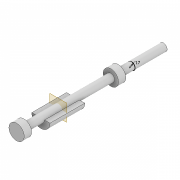
# Autodesk Inventor part: балансирный_вал
Saved by Autodesk Inventor 2021 (Build 250183000, 183)
## iProperties
Created: 2021-06-15
Part Number: балансирный_вал
Material: Типовые
Document SubType Name: Modeling
Designer: panda
Density: 1 g/cm^3
Appearance: По умолчанию
Mass: 101.736 g
Surface Area: 233.741 cm^2
Volume: 101.736 cm^3
Author: panda
Autodesk Inventor part; units mm, degrees
ref_plane "YZ Plane" through (0, 0, 0) normal (1, 0, 0) x (0, 1, 0)
ref_plane "XZ Plane" through (0, 0, 0) normal (0, 1, 0) x (-1, 0, 0)
ref_plane "XY Plane" through (0, 0, 0) normal (0, 0, 1) x (1, 0, 0)
sketch "Эскиз1" plane through (0, 0, 0) normal (0, 0, 1) x (1, 0, 0)
  circle A0 centre (0, 0) radius 8.5
  dimension "d1" = 17
  constraints: 1 centre point
  measures "d1" diameter of A0
extrude "Выдавливание1" add sketch "Эскиз1" against normal blind 55
sketch "Эскиз2" plane through (0, 0, 0) normal (0, 0, 1) x (1, 0, 0)
  circle A0 centre (0, 0) radius 8.5
  dimension "d10" = 17
  constraints: 1 centre point, 1 coincident
  measures "d10" diameter of A0
extrude "Выдавливание2" add sketch "Эскиз2" along normal blind 30
sketch "Эскиз3" plane through (0, 0, 30) normal (0, 0, 1) x (1, 0, 0)
  circle A0 centre (0, 0) radius 17.5
  dimension "d7" = 35
  constraints: 1 centre point, 1 coincident
  measures "d7" diameter of A0
extrude "Выдавливание3" add sketch "Эскиз3" along normal blind 17
sketch "Эскиз4" plane through (0, 0, 47) normal (0, 0, 1) x (1, 0, 0)
  circle A0 centre (0, 0) radius 8.5
  line L0 (8.5, 0) -> (20, 0) projected
  point P0 (-16, 0)
  dimension "d25" = 17
  constraints: 1 horizontal alignment, 1 other
extrude "Выдавливание4" add sketch "Эскиз4" along normal blind 15
sketch "Эскиз6" plane through (0, 0, 62) normal (0, 0, 1) x (1, 0, 0)
  circle A0 centre (0, 0) radius 8.5
  point P0 (-16, 0)
  point P1 (20, 0)
  dimension "d24" = 17
  constraints: 1 centre point
  measures "d24" diameter of A0
extrude "Выдавливание5" add sketch "Эскиз6" along normal blind 55
sketch "Эскиз7" plane through (0, 0, 117) normal (0, 0, 1) x (1, 0, 0)
  circle A0 centre (0, 0) radius 8.5
  dimension "d26" = 17
  constraints: 1 centre point, 1 coincident
  measures "d26" diameter of A0
extrude "Выдавливание6" add sketch "Эскиз7" along normal blind 130
sketch "Эскиз8" plane through (0, 0, 247) normal (0, 0, 1) x (1, 0, 0)
  circle A0 centre (0, 0) radius 17.5
  dimension "d23" = 35
  constraints: 1 centre point, 1 coincident
  measures "d23" diameter of A0
extrude "Выдавливание7" add sketch "Эскиз8" along normal blind 17
sketch "Эскиз9" plane through (0, 0, -55) normal (0, 0, -1) x (-1, 0, 0)
  circle A0 centre (0, 0) radius 8.5
  constraints: 1 centre point, 1 coincident
extrude "Выдавливание8" add sketch "Эскиз9" along normal blind 19.1
ref_plane "РабПлоскость1" through (0, 0, 168) normal (0, 0, 1) x (1, 0, 0)
sketch "Эскиз10" plane through (0, 0, 168) normal (0, 0, 1) x (1, 0, 0)
  circle A0 centre (0, 0) radius 8.5
  circle A1 centre (0, 0) radius 21
  line L0 (-21, 0) -> (21, 0)
  point P0 (-8.5, 0)
  point P1 (8.5, 0)
  dimension "d30" = 42
  constraints: 2 centre point, 2 coincident, 2 end point, 2 point on circle, 1 horizontal
  measures "d30" diameter of A1
extrude "Выдавливание9" add sketch "Эскиз10" along normal mid plane 80 contours L0 A1 A0 picked at (16.6299, -1.6752)
